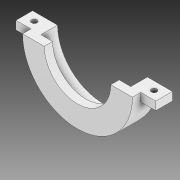
# Autodesk Inventor part: 22010B_Tube End Support_V2
Saved by Autodesk Inventor 2020 (Build 240168000, 168)
## iProperties
Created: 2019-11-08
Part Number: 22010B_Tube End Support_V2
Material: ABS Plastic
Document SubType Name: Modeling
Designer: RFLab
Density: 1.06 g/cm^3
Appearance: Smooth - White
Author: RFLab
Autodesk Inventor part; units mm, degrees
ref_plane "YZ Plane" through (0, 0, 0) normal (1, 0, 0) x (0, 1, 0)
ref_plane "XZ Plane" through (0, 0, 0) normal (0, 1, 0) x (-1, 0, 0)
ref_plane "XY Plane" through (0, 0, 0) normal (0, 0, 1) x (1, 0, 0)
sketch "Sketch1" plane through (0, 0, 0) normal (0, 0, 1) x (1, 0, 0)
  arc A0 (-33, 0) -> (33, 0) centre (0, 0) ccw
  arc A1 (-27, 0) -> (27, 0) centre (0, 0) ccw
  line L0 (-33, 0) -> (-27, 0)
  line L1 (27, 0) -> (33, 0)
  dimension "d0" = 66
  dimension "d1" = 54
  constraints: 4 end point, 4 point on circle, 2 centre point, 2 coincident, 2 horizontal
  measures "d0" diameter of A0
  measures "d1" diameter of A1
extrude "Extrusion1" add sketch "Sketch1" along normal blind 10
sketch "Sketch2" plane through (-33, 0, 0) normal (0, 1, 0) x (1, 0, 0)
  line L0 (6, 0) -> (6, -10) projected
  line L1 (6, 0) -> (-9, 0)
  line L2 (-9, 0) -> (-9, -10)
  line L3 (-9, -10) -> (6, -10)
  line L4 (6, -10) -> (6, 0)
  line L5 (66, 0) -> (60, 0) projected
  line L6 (60, 0) -> (75, 0)
  line L7 (75, 0) -> (75, -10)
  line L8 (75, -10) -> (60, -10)
  line L9 (60, -10) -> (60, 0)
  point P0 (33, 0)
  dimension "d4" = 15
  constraints: 16 end point, 4 parallel, 2 horizontal, 2 perpendicular, 1 collinear, 1 point on line
  measures "d4" distance of L0.start L1.end
extrude "Extrusion2" add sketch "Sketch2" against normal blind 5
sketch "Sketch3" plane through (-27, 0, 10) normal (0, 1, 0) x (1, 0, 0)
  circle A0 centre (-9, 5) radius 1.65
  circle A1 centre (63, 5) radius 1.65
  line L0 (0, 10) -> (-15, 10) projected
  line L1 (-15, 10) -> (-15, 0) projected
  line L2 (69, 10) -> (54, 10) projected
  line L3 (69, 0) -> (69, 10) projected
  point P0 (27, 10)
  dimension "d7" = 5
  dimension "d8" = 6
  dimension "d9" = 5
  dimension "d10" = 6
  dimension "d11" = 3.3
  constraints: 2 centre point, 1 equal radius
  measures "d7" distance from line of L0 A0.centre
  measures "d8" distance from line of L1 A0.centre
  measures "d9" distance from line of L2 A1.centre
  measures "d10" distance from line of L3 A1.centre
  measures "d11" diameter of A1
extrude "Extrusion3" cut sketch "Sketch3" against normal blind 5
sketch "Sketch4" plane through (0, 0, 10) normal (0, 0, 1) x (1, 0, 0)
  arc A0 (-33, 0) -> (33, 0) centre (0, 0) ccw
  arc A1 (-20, 0) -> (20, 0) centre (0, 0) ccw
  line L0 (-27, 0) -> (-42, 0) projected
  line L1 (33, 0) -> (20, 0)
  line L2 (-20, 0) -> (-33, 0)
  dimension "d14" = 40
  dimension "d15" = 66
  constraints: 4 end point, 4 point on circle, 2 centre point, 2 coincident, 1 point on line
  measures "d14" diameter of A1
  measures "d15" diameter of A0
extrude "Extrusion4" add sketch "Sketch4" along normal blind 5
body "Solid1"
